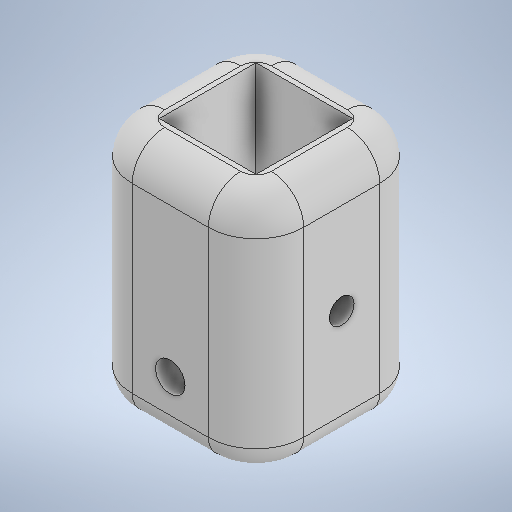
# Autodesk Inventor part: arm_collar
Saved by Autodesk Inventor 2025 (Build 290162000, 162)
## iProperties
Created: 2026-06-08
Part Number: arm_collar
Material: Generic
Document SubType Name: Modeling
Designer: localadmin
Density: 1 g/cm^3
Appearance: Default
Author: localadmin
Autodesk Inventor part; units mm, degrees
ref_plane "YZ Plane" through (0, 0, 0) normal (1, 0, 0) x (0, 1, 0)
ref_plane "XZ Plane" through (0, 0, 0) normal (0, 1, 0) x (-1, 0, 0)
ref_plane "XY Plane" through (0, 0, 0) normal (0, 0, 1) x (1, 0, 0)
sketch "Sketch1" plane through (0, 0, 0) normal (0, 0, 1) x (1, 0, 0)
  line L0 (0, 0) -> (36, 0)
  line L1 (36, 0) -> (36, 50)
  line L2 (36, 50) -> (0, 50)
  line L3 (0, 50) -> (0, 0)
  dimension "d0" = 36
  dimension "d1" = 50
  constraints: 8 end point, 2 parallel, 1 horizontal, 1 perpendicular
  measures "d0" distance of L0.start L0.end
  measures "d1" distance of L0.end L1.end
extrude "Extrusion1" add sketch "Sketch1" along normal mid plane 36
sketch "Sketch2" plane through (0, 50, 18) normal (0, 1, 0) x (1, 0, 0)
  line L0 (28.15, 7.85) -> (7.85, 7.85)
  line L1 (7.85, 7.85) -> (7.85, 28.15)
  line L2 (7.85, 28.15) -> (28.15, 28.15)
  line L3 (28.15, 28.15) -> (28.15, 7.85)
  line L4 (28.15, 7.85) -> (7.85, 28.15) construction
  line L5 (7.85, 7.85) -> (28.15, 28.15) construction
  line L6 (0, 36) -> (0, 0) projected
  point P0 (0, 18)
  point P1 (18, 18)
  point P2 (0, 18)
  dimension "d4" = 18
  dimension "d5" = 20.3
  dimension "d6" = 20.3
  constraints: 12 end point, 3 midpoint, 2 parallel, 1 horizontal, 1 perpendicular
  measures "d4" distance of point (0, 18) point (18, 18)
  measures "d5" distance of L0.end L1.end
  measures "d6" distance of L0.start L0.end
extrude "Extrusion2" cut sketch "Sketch2" against normal blind 33
sketch "Sketch3" plane through (0, 0, 18) normal (0, 0, 1) x (1, 0, 0)
  line L0 (0, 50) -> (0, 0) projected
  line L1 (0, 0) -> (36, 0) projected
  point P0 (18, 12)
  dimension "d9" = 18
  dimension "d10" = 12
  measures "d9" distance from line of point (18, 12) L0
  measures "d10" distance from line of L1 point (18, 12)
hole "Hole1" at (18, 12, 18) direction (0, 0, -1) diameter 6.2 end through all
sketch "Sketch8" plane through (7.85, 50, -10.15) normal (0, 0, 1) x (1, 0, 0)
  point P0 (-7.85, -50)
sketch "Sketch11" plane through (0, 0, 18) normal (-1, 0, 0) x (0, 0, 1)
  circle A0 centre (-18, 24) radius 2.6
  line L0 (0, 50) -> (0, 0) projected
  line L1 (-7.85, 17) -> (-28.15, 17) projected
  point P0 (-18, 0)
  dimension "d41" = 5.2
  dimension "d42" = 18
  dimension "d43" = 7
  constraints: 1 centre point
  measures "d41" diameter of A0
  measures "d42" distance from line of L0 A0.centre
  measures "d43" distance from line of L1 A0.centre
extrude "Extrusion6" cut sketch "Sketch11" against normal through all
fillet "Fillet1" radius 10 4 edges at (36, 25, 18) (0, 25, 18) (0, 25, -18) (36, 25, -18)
fillet "Fillet2" radius 5 8 edges at (18, 0, 18) (33.0711, 0, 15.0711) (36, 0, 0) (33.0711, 0, -15.0711) (18, 0, -18) (2.9289, 0, -15.0711) (0, 0, 0) (2.9289, 0, 15.0711)
fillet "Fillet3" radius 6.8 8 edges at (33.0711, 50, 15.0711) (18, 50, 18) (2.9289, 50, 15.0711) (0, 50, 0) (2.9289, 50, -15.0711) (18, 50, -18) (33.0711, 50, -15.0711) (36, 50, 0)
body "Solid1"
